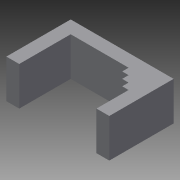
# Autodesk Inventor part: penHolderHolder
Saved by Autodesk Inventor 2013 SP2 (Build 170200200, 200)
## iProperties
Created: 2016-03-29
Part Number: penHolderHolder
Material: Generic
Document SubType Name: Modeling
Designer: 2016nfoss
Density: 1 g/cm^3
Author: 2016nfoss
Autodesk Inventor part; units mm, degrees
ref_plane "YZ Plane" through (0, 0, 0) normal (1, 0, 0) x (0, 1, 0)
ref_plane "XZ Plane" through (0, 0, 0) normal (0, 1, 0) x (-1, 0, 0)
ref_plane "XY Plane" through (0, 0, 0) normal (0, 0, 1) x (1, 0, 0)
sketch "Sketch1" plane through (0, 0, 0) normal (0, 1, 0) x (-1, 0, 0)
  line L0 (0, 0) -> (50.8, 0)
  line L1 (50.8, 0) -> (50.8, 31.75)
  line L2 (50.8, 31.75) -> (0, 31.75)
  line L3 (0, 31.75) -> (0, 0)
  line L4 (0, 0) -> (6.35, 0)
  line L5 (6.35, 0) -> (6.35, 6.35)
  line L6 (6.35, 6.35) -> (0, 6.35)
  line L7 (0, 6.35) -> (0, 0)
  line L8 (6.35, 6.35) -> (44.45, 6.35)
  line L9 (44.45, 6.35) -> (44.45, 31.75)
  line L10 (44.45, 31.75) -> (6.35, 31.75)
  line L11 (6.35, 31.75) -> (6.35, 6.35)
  line L12 (6.35, 6.35) -> (12.7, 6.35)
  line L13 (12.7, 6.35) -> (12.7, 12.7)
  line L14 (12.7, 12.7) -> (6.35, 12.7)
  line L15 (6.35, 12.7) -> (6.35, 6.35)
  line L16 (12.7, 6.35) -> (15.875, 6.35)
  line L17 (15.875, 6.35) -> (15.875, 9.525)
  line L18 (15.875, 9.525) -> (12.7, 9.525)
  line L19 (12.7, 9.525) -> (12.7, 6.35)
  line L20 (6.35, 12.7) -> (9.525, 12.7)
  line L21 (9.525, 12.7) -> (9.525, 15.875)
  line L22 (9.525, 15.875) -> (6.35, 15.875)
  line L23 (6.35, 15.875) -> (6.35, 12.7)
  dimension "d0" = 50.8
  dimension "d1" = 31.75
  dimension "d2" = 6.35
  dimension "d3" = 6.35
  dimension "d4" = 38.1
  dimension "d5" = 25.4
  dimension "d6" = 6.35
  dimension "d7" = 6.35
  dimension "d8" = 3.175
  dimension "d9" = 3.175
  dimension "d10" = 3.175
  dimension "d11" = 3.175
  constraints: 48 end point, 12 parallel, 6 horizontal, 6 perpendicular
  measures "d0" distance of L2.end L1.end
  measures "d1" distance of L1.end L0.end
  measures "d2" distance of L6.end L5.end
  measures "d3" distance of L5.end L4.end
  measures "d4" distance of L10.end L9.end
  measures "d5" distance of L9.end L8.end
  measures "d6" distance of L14.end L13.end
  measures "d7" distance of L13.end L12.end
  measures "d8" distance of L18.end L17.end
  measures "d9" distance of L17.end L16.end
  measures "d10" distance of L22.end L21.end
  measures "d11" distance of L21.end L20.end
extrude "Extrusion1" add sketch "Sketch1" along normal blind 19.05 contours L3 L6 L5 L0 | L5 L8 L9 L2 L1 L0 | L3 L2 L11 L6 | L11 L14 L13 L8 | L13 L18 L17 L8 | L11 L22 L21 L14
body "Solid1"
